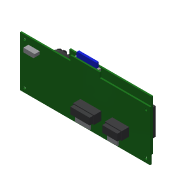
# Autodesk Inventor part: oledragu
Saved by Autodesk Inventor 2016 (Build 200138000, 138)
## iProperties
Created: 2016-03-29
Part Number: oledragu
Material: Generic
Document SubType Name: Modeling
Designer: admin
Density: 1 g/cm^3
Appearance: Default
Author: admin
Autodesk Inventor part; units mm, degrees
note: some values were not read from the file. Chosen so that the rebuilt part matches the saved one: copy form of "Circular Pattern1".
ref_plane "YZ Plane" through (0, 0, 0) normal (1, 0, 0) x (0, 1, 0)
ref_plane "XZ Plane" through (0, 0, 0) normal (0, 1, 0) x (-1, 0, 0)
sketch "Sketch1" plane through (0, 0, 0) normal (0, 1, 0) x (-1, 0, 0)
  line L0 (77.5, 30) -> (77.5, -30)
  line L1 (77.5, -30) -> (-77.5, -30)
  line L2 (-77.5, -30) -> (-77.5, 30)
  line L3 (-77.5, 30) -> (77.5, -30) construction
  line L4 (77.5, 30) -> (-77.5, -30) construction
  line L5 (-17.5, 30) -> (17.5, 30)
  line L6 (17.5, 30) -> (17.5, 36)
  line L7 (17.5, 36) -> (-17.5, 36)
  line L8 (-17.5, 36) -> (-17.5, 30)
  circle A0 centre (-72.5, 25) radius 1.6
  circle A1 centre (-72.5, -25) radius 1.6
  circle A2 centre (72.5, -25) radius 1.6
  circle A3 centre (72.5, 25) radius 1.6
  line L9 (-77.5, 30) -> (-17.5, 30)
  line L10 (17.5, 30) -> (77.5, 30)
  point P0 (0, 0)
  dimension "d0" = 155
  dimension "d1" = 60
  dimension "d4" = 6
  dimension "d5" = 35
  dimension "d6" = 60
  dimension "d7" = 3.2
  dimension "d9" = 5
  dimension "d10" = 3.2
  dimension "d11" = 3.2
  dimension "d12" = 3.2
  dimension "d13" = 5
  dimension "d15" = 5
  dimension "d16" = 5
  dimension "d17" = 5
  dimension "d18" = 5
  dimension "d19" = 5
  dimension "d20" = 5
  constraints: 22 end point, 5 parallel, 4 centre point, 3 horizontal, 3 perpendicular, 2 midpoint
  measures "d0" distance of L0.end L1.end
  measures "d1" distance of L0.start L0.end
  measures "d4" distance of L5.end L6.end
  measures "d5" distance between parallel lines of L6 L8
  measures "d6" distance between parallel lines of L8 L2
  measures "d7" diameter of A0
  measures "d9" distance from line of A0.centre L2
  measures "d10" diameter of A1
  measures "d11" diameter of A2
  measures "d12" diameter of A3
  measures "d13" distance from line of L0 A3.centre
  measures "d15" distance from line of L0 A2.centre
  measures "d16" distance from line of L1 A2.centre
  measures "d17" distance from line of L1 A1.centre
  measures "d18" distance from line of L2 A1.centre
  measures "d19" distance from line of L9 A0.centre
  measures "d20" distance from line of L10 A3.centre
extrude "Extrusion1" add sketch "Sketch1" along normal blind 1.8
ref_plane "Work Plane1" through (0, 11.8, 0) normal (0, 1, 0) x (1, 0, 0)
sketch "Sketch2" plane through (0, 11.8, 0) normal (0, 1, 0) x (1, 0, 0)
  line L0 (67.5, 30) -> (-30.5, 30)
  line L1 (-30.5, 30) -> (-30.5, -30)
  line L2 (-30.5, -30) -> (67.5, -30)
  line L3 (67.5, -30) -> (67.5, 30)
  point P0 (0, 0)
  dimension "d23" = 98
  constraints: 8 end point, 2 parallel, 1 horizontal, 1 perpendicular
  measures "d23" distance between parallel lines of L3 L1
extrude "Extrusion2" add sketch "Sketch2" along normal blind 1.8
sketch "Sketch3" plane through (0, 1.8, 0) normal (0, 1, 0) x (1, 0, 0)
  line L0 (-54, 6.25) -> (-41, 6.25)
  line L1 (-41, 6.25) -> (-41, -6.25)
  line L2 (-41, -6.25) -> (-54, -6.25)
  line L3 (-54, -6.25) -> (-54, 6.25)
  line L4 (-54, 6.25) -> (-41, -6.25) construction
  line L5 (-41, 6.25) -> (-54, -6.25) construction
  line L6 (77.5, 30) -> (-77.5, 30) projected
  line L7 (-77.5, 30) -> (-77.5, -30) projected
  point P0 (0, 0)
  point P1 (-47.5, 0)
  dimension "d26" = 13
  dimension "d27" = 12.5
  dimension "d30" = 30
  dimension "d31" = 30
  constraints: 12 end point, 2 midpoint, 2 parallel, 1 horizontal, 1 perpendicular
  measures "d26" distance of L1.end L2.end
  measures "d27" distance of L0.end L1.end
  measures "d30" distance from line of L6 point (-47.5, 0)
  measures "d31" distance from line of L7 point (-47.5, 0)
extrude "Extrusion3" add sketch "Sketch3" along normal blind 6
sketch "Sketch4" plane through (0, 7.8, 0) normal (0, 1, 0) x (1, 0, 0)
  line L0 (-41, 6.25) -> (-54, 6.25) projected
  line L1 (-54, -6.25) -> (-41, -6.25) projected
  line L2 (-47.5, 6.25) -> (-47.5, -6.25)
  circle A0 centre (-47.5, 0) radius 3
  point P0 (0, 0)
  dimension "d32" = 6
  constraints: 3 midpoint, 2 end point, 1 centre point
  measures "d32" diameter of A0
extrude "Extrusion4" add sketch "Sketch4" along normal blind 17
sketch "Sketch5" plane through (-47.5, 24.8, 0) normal (0, 1, 0) x (1, 0, 0)
  circle A0 centre (0, 0) radius 3 projected
  circle A1 centre (0, 0) radius 15
  point P0 (47.5, 0)
  dimension "d35" = 30
  constraints: 1 centre point, 1 coincident
  measures "d35" diameter of A1
extrude "Extrusion5" add sketch "Sketch5" against normal blind 8.5 separate body contours A0 | A1
sketch "Sketch6" plane through (0, 1.8, 0) normal (0, 1, 0) x (1, 0, 0)
  line L0 (-17.5, -30) -> (-17.5, -36) projected
  line L1 (-17.5, -36) -> (17.5, -36) projected
  line L2 (-14.25, -36) -> (14.25, -36)
  line L3 (14.25, -36) -> (14.25, -6)
  line L4 (14.25, -6) -> (-14.25, -6)
  line L5 (-14.25, -6) -> (-14.25, -36)
  point P0 (0, 0)
  dimension "d38" = 28.5
  dimension "d39" = 30
  dimension "d40" = 3.25
  constraints: 8 end point, 2 parallel, 1 horizontal, 1 perpendicular, 1 point on line
  measures "d38" distance of L4.end L3.end
  measures "d39" distance of L3.end L2.end
  measures "d40" distance between parallel lines of L0 L5
extrude "Extrusion6" add sketch "Sketch6" along normal blind 3 separate body
chamfer "Chamfer1" distance 4 angle 45 1 edges at (-62.5, 24.8, 0)
fillet "Fillet1" radius 6 2 edges at (-58.5, 24.8, 0) (-62.5, 20.8, 0)
sketch "Sketch7" plane through (-47.5, 24.8, 0) normal (0, 1, 0) x (1, 0, 0)
  circle A0 centre (0, 0) radius 8.5147 projected
  line L0 (1, 14.9666) -> (1, 7)
  line L1 (1, 7) -> (-1, 7)
  line L2 (-1, 7) -> (-1, 14.9666)
  circle A1 centre (0, 0) radius 15
  point P0 (47.5, 0)
  constraints: 6 end point, 2 point on circle, 1 centre point, 1 coincident, 1 parallel
extrude "Extrusion7" add sketch "Sketch7" against normal up to next contours L0 L1 L2 A0 | A0 L2 A1 L0 picked at (-0.1113, 7.5027) picked at (-0.778, 10.6435) bodies 2
pattern_circular "Circular Pattern1" count 14 over 360 about axis through (-47.5, 18.8, 0) along (0, -1, 0) of "Extrusion7" geometry pattern yes bodies 2
fillet "Fillet2" radius 3 14 edges at (-54.0083, 24.8, 13.5145) (-59.2275, 24.8, 9.3523) (-62.1239, 24.8, 3.3378) (-62.1239, 24.8, -3.3378) (-59.2275, 24.8, -9.3523) (-54.0083, 24.8, -13.5145) (-47.5, 24.8, -15) (-40.9917, 24.8, -13.5145) (-35.7725, 24.8, -9.3523) (-32.8761, 24.8, -3.3378) (-32.8761, 24.8, 3.3378) (-35.7725, 24.8, 9.3523) (-40.9917, 24.8, 13.5145) (-47.5, 24.8, 15)
sketch "Sketch8" plane through (0, 13.6, 0) normal (0, 1, 0) x (1, 0, 0)
  line L0 (-30.5, 30) -> (-30.5, -30) projected
  line L1 (-28.5, 16) -> (65.5, 16)
  line L2 (65.5, 16) -> (65.5, -16)
  line L3 (65.5, -16) -> (-28.5, -16)
  line L4 (-28.5, -16) -> (-28.5, 16)
  line L5 (-28.5, 16) -> (65.5, -16) construction
  line L6 (65.5, 16) -> (-28.5, -16) construction
  point P0 (0, 0)
  point P1 (18.5, 0)
  dimension "d58" = 94
  dimension "d59" = 32
  dimension "d60" = 2
  constraints: 12 end point, 2 midpoint, 2 parallel, 1 horizontal, 1 perpendicular
  measures "d58" distance between parallel lines of L2 L4
  measures "d59" distance between parallel lines of L3 L1
  measures "d60" distance between parallel lines of L0 L4
sketch "Sketch9" plane through (-14.25, 1.8, 36) normal (0, 0, 1) x (1, 0, 0)
  line L0 (0, 0) -> (28.5, 0) projected
  line L1 (0, 0) -> (0, 3) projected
  line L2 (2.25, 0) -> (26.25, 0)
  line L3 (26.25, 0) -> (26.25, 2.5)
  line L4 (26.25, 2.5) -> (2.25, 2.5)
  line L5 (2.25, 2.5) -> (2.25, 0)
  point P0 (14.25, -1.8)
  dimension "d53" = 24
  dimension "d54" = 2.5
  dimension "d55" = 2.25
  constraints: 8 end point, 2 parallel, 1 horizontal, 1 perpendicular, 1 point on line
  measures "d53" distance of L4.end L3.end
  measures "d54" distance of L3.end L2.end
  measures "d55" distance between parallel lines of L1 L5
extrude "Extrusion8" add sketch "Sketch9" along normal blind 6 and the other way blind 10 separate body
extrude "Extrusion9" add sketch "Sketch8" along normal blind 5 separate body
sketch "Sketch10" plane through (0, 18.6, 0) normal (0, 1, 0) x (1, 0, 0)
  line L0 (-28.5, 16) -> (-28.5, -16) projected
  line L1 (-20, 12.1925) -> (57, 12.1925)
  line L2 (57, 12.1925) -> (57, -12.8075)
  line L3 (57, -12.8075) -> (-20, -12.8075)
  line L4 (-20, -12.8075) -> (-20, 12.1925)
  point P0 (0, 0)
  dimension "d63" = 77
  dimension "d64" = 25
  dimension "d65" = 8.5
  constraints: 8 end point, 2 parallel, 1 horizontal, 1 perpendicular
  measures "d63" distance between parallel lines of L2 L4
  measures "d64" distance between parallel lines of L3 L1
  measures "d65" distance between parallel lines of L0 L4
extrude "Extrusion10" cut sketch "Sketch10" against normal blind 0.5 bodies 5
sketch "Sketch11" plane through (-47.5, 24.8, 0) normal (0, 1, 0) x (1, 0, 0)
  circle A0 centre (0, 0) radius 3 projected
  point P0 (47.5, 0)
extrude "Extrusion11" cut sketch "Sketch11" against normal blind 1 bodies 1
sketch "Sketch12" plane through (0, 4.8, 0) normal (0, 1, 0) x (1, 0, 0)
  line L0 (-14.25, -36) -> (14.25, -36) projected
  circle A0 centre (0, -36) radius 10
  point P0 (0, 0)
  dimension "d72" = 20
  constraints: 1 centre point, 1 midpoint
  measures "d72" diameter of A0
extrude "Extrusion12" cut sketch "Sketch12" against normal blind 2.5 bodies 3
fillet "Fillet3" radius 1 2 edges at (10, 3.55, 36) (-10, 3.55, 36)
sketch "Sketch13" plane through (-12, 4.3, 42) normal (0, 1, 0) x (1, 0, 0)
  line L0 (0, 16) -> (0, 0) projected
  line L1 (24, 0) -> (0, 0) projected
  line L2 (24, 16) -> (24, 0) projected
  line L3 (4, 3) -> (20, 3)
  line L4 (21, 4) -> (21, 10.1)
  line L5 (20, 11.1) -> (4, 11.1)
  line L6 (3, 10.1) -> (3, 4)
  arc A0 (3, 4) -> (4, 3) centre (4, 4) ccw
  arc A1 (20, 3) -> (21, 4) centre (20, 4) ccw
  line L7 (3, 7) -> (21, 7)
  line L8 (3, 7.1) -> (21, 7.1)
  arc A2 (4, 11.1) -> (3, 10.1) centre (4, 10.1) ccw
  arc A3 (21, 10.1) -> (20, 11.1) centre (20, 10.1) ccw
  point P0 (12, 42)
  point P1 (21, 11.1)
  point P2 (3, 11.1)
  dimension "d76" = 3
  dimension "d77" = 3
  dimension "d78" = 3
  dimension "d79" = 1
  dimension "d80" = 0.1
  dimension "d81" = 4
  dimension "d84" = 4
  dimension "d85" = 1
  constraints: 12 end point, 8 point on circle, 8 point on line, 8 tangent, 4 centre point, 3 perpendicular, 2 equal radius, 2 parallel, 1 horizontal
  measures "d76" distance between parallel lines of L1 L3
  measures "d77" distance between parallel lines of L2 L4
  measures "d78" distance between parallel lines of L0 L6
  measures "d79" radius of A0
  measures "d80" distance between parallel lines of L8 L7
  measures "d81" distance between parallel lines of L3 L7
  measures "d84" distance between parallel lines of L8 L5
  measures "d85" radius of A2
extrude "Extrusion13" cut sketch "Sketch13" against normal blind 0.1 contours A0 L6 L7 L4 A1 L3 | L6 A2 L5 A3 L4 L8 bodies 4
fillet "Fillet4" radius 1 2 edges at (12, 3.05, 42) (-12, 3.05, 42)
sketch "Sketch15" plane through (0, 0, 0) normal (0, -1, 0) x (1, 0, 0)
  line L0 (77.5, -30) -> (-77.5, -30) projected
  line L1 (32.5, -3) -> (52.5, -3)
  line L2 (52.5, -3) -> (52.5, -13)
  line L3 (52.5, -13) -> (32.5, -13)
  line L4 (32.5, -13) -> (32.5, -3)
  line L5 (-5.5, -3) -> (19.5, -3)
  line L6 (19.5, -3) -> (19.5, -13)
  line L7 (19.5, -13) -> (-5.5, -13)
  line L8 (-5.5, -13) -> (-5.5, -3)
  line L9 (77.5, 30) -> (77.5, -30) projected
  point P0 (0, 0)
  dimension "d92" = 17
  dimension "d93" = 10
  dimension "d95" = 17
  dimension "d96" = 10
  dimension "d97" = 20
  dimension "d98" = 25
  dimension "d115" = 25
  dimension "d116" = 83
  constraints: 16 end point, 4 parallel, 2 horizontal, 2 perpendicular
  measures "d92" distance between parallel lines of L0 L3
  measures "d93" distance between parallel lines of L1 L3
  measures "d95" distance between parallel lines of L0 L7
  measures "d96" distance between parallel lines of L5 L7
  measures "d97" distance between parallel lines of L2 L4
  measures "d98" distance between parallel lines of L6 L8
  measures "d115" distance between parallel lines of L9 L2
  measures "d116" distance between parallel lines of L9 L8
extrude "Extrusion14" add sketch "Sketch15" along normal blind 13 separate body
sketch "Sketch16" plane through (52.5, 0, -13) normal (0, 0, -1) x (-1, 0, 0)
  line L0 (0, 0) -> (20, 0) projected
  line L1 (0, 0) -> (0, -13) projected
  line L2 (20, 0) -> (20, -13) projected
  line L3 (33, 0) -> (58, 0) projected
  line L4 (33, 0) -> (33, -13) projected
  line L5 (58, -13) -> (33, -13) projected
  line L6 (58, 0) -> (58, -13) projected
  line L7 (37, -9.5) -> (54, -9.5) construction
  line L8 (37, -8.8) -> (54, -8.8)
  line L9 (54, -10.2) -> (37, -10.2)
  arc A0 (37, -8.8) -> (37, -10.2) centre (37, -9.5) ccw
  arc A1 (54, -10.2) -> (54, -8.8) centre (54, -9.5) ccw
  line L10 (4, -9.5) -> (16, -9.5) construction
  line L11 (4, -8.8) -> (16, -8.8)
  line L12 (16, -10.2) -> (4, -10.2)
  arc A2 (4, -8.8) -> (4, -10.2) centre (4, -9.5) ccw
  arc A3 (16, -10.2) -> (16, -8.8) centre (16, -9.5) ccw
  point P0 (52.5, 0)
  point P1 (45.5, -9.5)
  point P2 (10, -9.5)
  dimension "d101" = 10.2
  dimension "d102" = 10.2
  dimension "d103" = 1.4
  dimension "d104" = 1.4
  dimension "d105" = 4
  dimension "d106" = 4
  dimension "d107" = 4
  dimension "d108" = 4
  constraints: 16 end point, 8 point on circle, 8 tangent, 4 centre point, 2 midpoint, 2 parallel, 1 perpendicular
  measures "d101" distance between parallel lines of L0 L12
  measures "d102" distance between parallel lines of L3 L9
  measures "d103" distance between parallel lines of L8 L9
  measures "d104" distance between parallel lines of L11 L12
  measures "d105" distance from line of L4 L7.start
  measures "d106" distance from line of L6 L7.end
  measures "d107" distance from line of L1 L10.start
  measures "d108" distance from line of L2 L10.end
extrude "Extrusion15" add sketch "Sketch16" along normal mid plane 13 separate body contours L8 A1 L9 A0 | L11 A3 L12 A2
sketch "Sketch17" plane through (0, -13, 0) normal (0, -1, 0) x (1, 0, 0)
  line L0 (52.5, -3) -> (32.5, -3) projected
  line L1 (32.5, -3) -> (32.5, -13) projected
  line L2 (32.5, -13) -> (52.5, -13) projected
  line L3 (52.5, -13) -> (52.5, -3) projected
  line L4 (33.5, -4) -> (51.5, -4)
  line L5 (51.5, -4) -> (51.5, -12)
  line L6 (51.5, -12) -> (33.5, -12)
  line L7 (33.5, -12) -> (33.5, -4)
  line L8 (19.5, -3) -> (-5.5, -3) projected
  line L9 (-5.5, -3) -> (-5.5, -13) projected
  line L10 (-5.5, -13) -> (19.5, -13) projected
  line L11 (19.5, -13) -> (19.5, -3) projected
  line L12 (-4.5, -4) -> (18.5, -4)
  line L13 (18.5, -4) -> (18.5, -12)
  line L14 (18.5, -12) -> (-4.5, -12)
  line L15 (-4.5, -12) -> (-4.5, -4)
  point P0 (0, 0)
  dimension "d111" = 1
  dimension "d112" = 1
  constraints: 16 end point, 6 other
  measures "d111" distance between parallel lines of L3 L5
  measures "d112" distance between parallel lines of L8 L12
extrude "Extrusion16" cut sketch "Sketch17" against normal up to surface (4.2 mm away) bodies 6
sketch "Sketch18" plane through (0, 0, 0) normal (0, -1, 0) x (1, 0, 0)
  line L0 (-77.5, 30) -> (-17.5, 30) projected
  line L1 (-77.5, -30) -> (-77.5, 30) projected
  line L2 (-67.5, 22) -> (-54, 22)
  line L3 (-54, 22) -> (-54, 18.5)
  line L4 (-55.5, 17) -> (-67.5, 17)
  line L5 (-67.5, 17) -> (-67.5, 22)
  line L6 (-54, 18.5) -> (-55.5, 17)
  line L7 (-85, 51.4982) -> (6.0709, 51.4982) construction
  line L8 (6.0709, 51.4982) -> (6.0709, -35.073) construction
  line L9 (6.0709, -35.073) -> (-85, -35.073) construction
  line L10 (-85, -35.073) -> (-85, 51.4982) construction
  point P0 (0, 0)
  dimension "d117" = 1.5
  dimension "d118" = 5
  dimension "d119" = 13.5
  dimension "d120" = 135
  dimension "d121" = 8
  dimension "d122" = 10
  constraints: 10 end point, 2 parallel, 1 horizontal, 1 perpendicular, 2 other
  measures "d117" horizontal distance of L3.end L4.start
  measures "d118" distance between parallel lines of L4 L2
  measures "d119" distance between parallel lines of L5 L3
  measures "d120" angle of L3 L6
  measures "d121" distance between parallel lines of L0 L2
  measures "d122" distance between parallel lines of L1 L5
extrude "Extrusion17" add sketch "Sketch18" along normal blind 6 separate body
body "Solid1"
body "Solid2"
body "Solid3"
body "Solid4"
body "Solid5"
body "Solid6"
body "Solid7"
body "Solid8"
